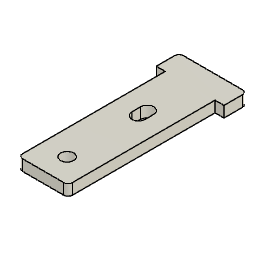
bat case v3 (Autodesk Fusion 360 design; units mm, degrees)
Autodesk Fusion 360 part; units mm, degrees
sketch "Sketch1" plane through (0, 0, 0) normal (0, 0, 1) x (1, 0, 0)
  line L0 (69.8497, 48.3293) -> (69.8497, 19.9293)
  line L1 (69.8497, 19.9293) -> (58.4497, 19.9293)
  line L2 (58.4497, 19.9293) -> (58.4497, 48.3293)
  line L3 (56.3997, 53.5293) -> (71.8997, 53.5293)
  line L4 (71.8997, 53.5293) -> (71.8997, 48.3293)
  line L5 (56.3997, 48.3293) -> (56.3997, 53.5293)
  line L6 (64.1497, 19.9293) -> (64.1497, 23.9293) construction
  circle A0 centre (64.1497, 25.4293) radius 1.5
  line L7 (64.1497, 26.9293) -> (64.1497, 40.2293) construction
  line L8 (65.6497, 41.7293) -> (65.6497, 43.7293)
  arc A1 (65.6497, 43.7293) -> (62.6497, 43.7293) centre (64.1497, 43.7293) ccw
  line L9 (62.6497, 43.7293) -> (62.6497, 41.7293)
  arc A2 (62.6497, 41.7293) -> (65.6497, 41.7293) centre (64.1497, 41.7293) ccw
  line L10 (64.1497, 40.2293) -> (64.1497, 45.2293) construction
  line L11 (58.4497, 53.5293) -> (69.8497, 53.5293)
  line L12 (71.8997, 53.5293) -> (64.1497, 53.5293) construction
  line L13 (69.8497, 53.5293) -> (64.1497, 53.5293) construction
  line L14 (56.3997, 48.3293) -> (58.4497, 48.3293)
  line L15 (69.8497, 48.3293) -> (71.8997, 48.3293)
  dimension "d1" = 11.4
  dimension "d2" = 33.6
  dimension "d3" = 15.5
  dimension "d4" = 5.2
  dimension "d5" = 4
  dimension "d7" = 3
  dimension "d8" = 13.3
  dimension "d9" = 3
  constraint vertical L0
  constraint horizontal L1
  constraint vertical L2
  constraint horizontal L3
  constraint vertical L4
  constraint vertical L5
  constraint midpoint L1 L6.start
  constraint perpendicular L1 L6
  constraint coincident L6.end A0
  constraint coincident A0 L7.start
  constraint vertical L7
  constraint tangent L8 A1
  constraint tangent A1 L9
  constraint parallel L8 L9
  constraint tangent L9 A2
  constraint tangent L8 A2
  constraint midpoint L7.end A2
  constraint midpoint A1 L10.end
  constraint parallel L7 L10
  constraint perpendicular L0 L11
  constraint perpendicular L4 L14
  constraint midpoint L3 L12.end
  constraint midpoint L11 L12.end
  constraint coincident L0.start L14
  constraint collinear L14 L15
  measures "d1" distance of L11.start L11.end
  measures "d2" distance of L11.start L1.end
  measures "d3" distance of L3.start L3.end
  measures "d4" distance of L3.start L5.start
  measures "d5" distance of L6.start L6.end
  measures "d7" diameter of A0
  measures "d8" distance of L7.start L7.end
  measures "d9" diameter of A1
extrude "Extrude1" add sketch "Sketch1" along normal blind 2.5
fillet "Fillet1" radius 1 2 edges at (56.3997, 53.5293, 1.25) (71.8997, 53.5293, 1.25)
fillet "Fillet2" radius 1 2 edges at (69.8497, 19.9293, 1.25) (58.4497, 19.9293, 1.25)
